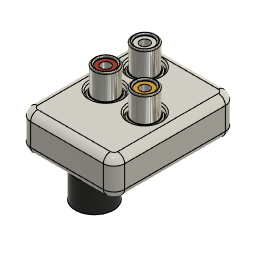
AV Adapter case v11 (Autodesk Fusion 360 design; units mm, degrees)
Autodesk Fusion 360 part; units mm, degrees
sketch "top place" plane through (0, 0, 0) normal (0, 0, 1) x (1, 0, 0) in component "PCB"
  arc A0 (28, 37) -> (27, 38) centre (27, 37) ccw
  line L0 (28, 37) -> (28, 1)
  line L1 (1, 38) -> (27, 38)
  arc A1 (27, 0) -> (28, 1) centre (27, 1) ccw
  line L2 (27, 0) -> (1, 0)
  arc A2 (0, 1) -> (1, 0) centre (1, 1) ccw
  line L3 (0, 1) -> (0, 37)
  arc A3 (1, 38) -> (0, 37) centre (1, 37) ccw
  arc A4 (25.3133, 15.5251) -> (25.3133, 20.4749) centre (21, 18) ccw
  circle A5 centre (7, 32) radius 1.7
  arc A6 (23.4749, 22.3133) -> (18.5251, 22.3133) centre (21, 18) ccw
  arc A7 (3.4645, 34.2627) -> (3.4645, 29.7373) centre (7, 32) ccw
  circle A8 centre (21, 18) radius 3.1
  arc A9 (23.2627, 21.5355) -> (18.7373, 21.5355) centre (21, 18) ccw
  arc A10 (11.3133, 29.5251) -> (11.3133, 34.4749) centre (7, 32) ccw
  arc A11 (16.6867, 20.4749) -> (16.6867, 15.5251) centre (21, 18) ccw
  arc A12 (24.5355, 15.7373) -> (24.5355, 20.2627) centre (21, 18) ccw
  arc A13 (18.5251, 13.6867) -> (23.4749, 13.6867) centre (21, 18) ccw
  arc A14 (4.5251, 27.6867) -> (9.4749, 27.6867) centre (7, 32) ccw
  arc A15 (9.4749, 36.3133) -> (4.5251, 36.3133) centre (7, 32) ccw
  arc A16 (4.7373, 28.4645) -> (9.2627, 28.4645) centre (7, 32) ccw
  circle A17 centre (7, 18) radius 3.1
  arc A18 (11.3133, 15.5251) -> (11.3133, 20.4749) centre (7, 18) ccw
  arc A19 (9.2627, 35.5355) -> (4.7373, 35.5355) centre (7, 32) ccw
  arc A20 (4.5251, 13.6867) -> (9.4749, 13.6867) centre (7, 18) ccw
  arc A21 (2.6867, 34.4749) -> (2.6867, 29.5251) centre (7, 32) ccw
  arc A22 (4.7373, 14.4645) -> (9.2627, 14.4645) centre (7, 18) ccw
  arc A23 (10.5355, 29.7373) -> (10.5355, 34.2627) centre (7, 32) ccw
  arc A24 (18.7373, 14.4645) -> (23.2627, 14.4645) centre (21, 18) ccw
  arc A25 (3.4645, 20.2627) -> (3.4645, 15.7373) centre (7, 18) ccw
  circle A26 centre (7, 32) radius 3.1
  arc A27 (17.4645, 20.2627) -> (17.4645, 15.7373) centre (21, 18) ccw
  circle A28 centre (21, 18) radius 1.7
  circle A29 centre (7, 18) radius 1.7
  arc A30 (9.2627, 21.5355) -> (4.7373, 21.5355) centre (7, 18) ccw
  arc A31 (9.4749, 22.3133) -> (4.5251, 22.3133) centre (7, 18) ccw
  arc A32 (2.6867, 20.4749) -> (2.6867, 15.5251) centre (7, 18) ccw
  arc A33 (10.5355, 15.7373) -> (10.5355, 20.2627) centre (7, 18) ccw
  arc A34 (4.7373, 21.5355) -> (3.4645, 20.2627) centre (7, 18) ccw
  arc A35 (10.5355, 20.2627) -> (9.2627, 21.5355) centre (7, 18) ccw
  arc A36 (17.4645, 15.7373) -> (18.7373, 14.4645) centre (21, 18) ccw
  arc A37 (9.4749, 27.6867) -> (11.3133, 29.5251) centre (7, 32) ccw
  arc A38 (25.3133, 20.4749) -> (23.4749, 22.3133) centre (21, 18) ccw
  arc A39 (4.7373, 35.5355) -> (3.4645, 34.2627) centre (7, 32) ccw
  arc A40 (16.6867, 15.5251) -> (18.5251, 13.6867) centre (21, 18) ccw
  arc A41 (9.2627, 14.4645) -> (10.5355, 15.7373) centre (7, 18) ccw
  arc A42 (2.6867, 29.5251) -> (4.5251, 27.6867) centre (7, 32) ccw
  arc A43 (23.4749, 13.6867) -> (25.3133, 15.5251) centre (21, 18) ccw
  arc A44 (18.5251, 22.3133) -> (16.6867, 20.4749) centre (21, 18) ccw
  arc A45 (4.5251, 22.3133) -> (2.6867, 20.4749) centre (7, 18) ccw
  arc A46 (3.4645, 29.7373) -> (4.7373, 28.4645) centre (7, 32) ccw
  arc A47 (18.7373, 21.5355) -> (17.4645, 20.2627) centre (21, 18) ccw
  arc A48 (23.2627, 14.4645) -> (24.5355, 15.7373) centre (21, 18) ccw
  arc A49 (11.3133, 20.4749) -> (9.4749, 22.3133) centre (7, 18) ccw
  arc A50 (9.2627, 28.4645) -> (10.5355, 29.7373) centre (7, 32) ccw
  arc A51 (10.5355, 34.2627) -> (9.2627, 35.5355) centre (7, 32) ccw
  arc A52 (9.4749, 13.6867) -> (11.3133, 15.5251) centre (7, 18) ccw
  arc A53 (11.3133, 34.4749) -> (9.4749, 36.3133) centre (7, 32) ccw
  arc A54 (2.6867, 15.5251) -> (4.5251, 13.6867) centre (7, 18) ccw
  arc A55 (24.5355, 20.2627) -> (23.2627, 21.5355) centre (21, 18) ccw
  arc A56 (4.5251, 36.3133) -> (2.6867, 34.4749) centre (7, 32) ccw
  arc A57 (3.4645, 15.7373) -> (4.7373, 14.4645) centre (7, 18) ccw
extrude "Extrude1" add sketch "top place" against normal blind 1.6 contours A0 L0 L1 A1 L2 A2 L3 A3 | A4 A6 A11 A13 A38 A40 A43 A44 | A5 | A7 A16 A19 A23 A39 A46 A50 A51 | A8 | A9 A12 A24 A27 A36 A47 A48 A55 | A10 A14 A15 A21 A37 A42 A53 A56 | A17 | A18 A20 A31 A32 A45 A49 A52 A54 | A22 A25 A30 A33 A34 A35 A41 A57 | A26 | A28 | A29 makes body 1 in component "PCB"
extrude "Extrude2" add sketch "top place" along normal blind 16.3 contours A8 | A17 | A26 bodies 1 in component "PCB"
extrude "Extrude3" add sketch "top place" along normal blind 17 contours A7 A16 A19 A23 A39 A46 A50 A51 | A9 A12 A24 A27 A36 A47 A48 A55 | A22 A25 A30 A33 A34 A35 A41 A57 bodies 1 in component "PCB"
extrude "Extrude4" add sketch "top place" along normal blind 8 contours A4 A6 A11 A13 A38 A40 A43 A44 | A10 A14 A15 A21 A37 A42 A53 A56 | A18 A20 A31 A32 A45 A49 A52 A54 bodies 1 in component "PCB"
fillet "Fillet2" radius 0.5 9 edges at (10.1265, 21.8671, 8) (9.478, 21.3881, 17) (4.1098, 19.121, 17) (10.8671, 28.8735, 8) (4.522, 28.6119, 17) (4.1098, 33.121, 17) (24.8671, 14.8735, 8) (18.522, 14.6119, 17) (18.1098, 19.121, 17) on bodies 1 in component "PCB"
ref_plane "WorkPlane1" through (0, 0, -1.6) normal (0, 0, 1) x (1, 0, 0) in component "PCB"
sketch "bottom place" plane through (0, 0, -1.6) normal (0, 0, 1) x (1, 0, 0) in component "PCB"
  arc A0 (28, 37) -> (27, 38) centre (27, 37) ccw
  line L0 (27, 0) -> (1, 0)
  arc A1 (27, 0) -> (28, 1) centre (27, 1) ccw
  arc A2 (0, 1) -> (1, 0) centre (1, 1) ccw
  line L1 (0, 1) -> (0, 37)
  line L2 (28, 37) -> (28, 1)
  arc A3 (1, 38) -> (0, 37) centre (1, 37) ccw
  line L3 (1, 38) -> (27, 38)
  circle A4 centre (13, 8) radius 6.8
  arc A5 (11.9, 14.1) -> (14.1, 14.1) centre (13, 14.2) ccw
  circle A6 centre (13, 8) radius 6.2
  circle A7 centre (16.5, 8) radius 0.8
  circle A8 centre (9.5, 8) radius 0.8
  circle A9 centre (15.47, 5.53) radius 0.8
  circle A10 centre (13, 4.5) radius 0.8
  circle A11 centre (10.53, 5.53) radius 0.8
extrude "Extrude5" add sketch "bottom place" against normal blind 14.51 contours A7 | A8 | A9 | A10 | A11 bodies 1 in component "PCB"
chamfer "Chamfer1" distance 0.5 angle 45 5 edges at (15.7541, 8.2893, -16.11) (14.7241, 5.8193, -16.11) (12.2541, 4.7893, -16.11) (9.7841, 5.8193, -16.11) (8.7541, 8.2893, -16.11) on bodies 1 in component "PCB"
extrude "Extrude6" add sketch "bottom place" against normal blind 3 from surface at -3 contours A5 A6 | A5 A6 bodies 1 in component "PCB"
extrude "Extrude7" add sketch "bottom place" against normal blind 10 from surface at -5.5 contours A4 bodies 1 in component "PCB"
sketch "bottom stop mask" plane through (0, 0, -1.6) normal (0, 0, 1) x (1, 0, 0) in component "PCB"
  line L0 (27, 0) -> (1, 0)
  arc A0 (27, 0) -> (28, 1) centre (27, 1) ccw
  line L1 (0, 1) -> (0, 37)
  arc A1 (28, 37) -> (27, 38) centre (27, 37) ccw
  line L2 (1, 38) -> (27, 38)
  arc A2 (1, 38) -> (0, 37) centre (1, 37) ccw
  line L3 (28, 37) -> (28, 1)
  arc A3 (0, 1) -> (1, 0) centre (1, 1) ccw
  line L4 (14.5294, 4.5894) -> (16.4106, 2.7082)
  circle A4 centre (24.5355, 21.5355) radius 1.3716
  arc A5 (16.4106, 2.7082) -> (18.2918, 4.5894) centre (17.3512, 3.6488) ccw
  line L5 (9.5, 9.3302) -> (6.8396, 9.3302)
  arc A6 (16.5, 9.3302) -> (16.5, 6.6698) centre (16.5, 8) ccw
  arc A7 (9.5, 6.6698) -> (9.5, 9.3302) centre (9.5, 8) ccw
  line L6 (14.3302, 1.8396) -> (14.3302, 4.5)
  line L7 (16.5, 6.6698) -> (19.1604, 6.6698)
  circle A8 centre (17.4645, 21.5355) radius 1.3716
  circle A9 centre (24.5355, 14.4645) radius 1.3716
  arc A10 (19.1604, 6.6698) -> (19.1604, 9.3302) centre (19.1604, 8) ccw
  line L8 (11.6698, 4.5) -> (11.6698, 1.8396)
  line L9 (6.8396, 6.6698) -> (9.5, 6.6698)
  line L10 (19.1604, 9.3302) -> (16.5, 9.3302)
  arc A11 (6.8396, 9.3302) -> (6.8396, 6.6698) centre (6.8396, 8) ccw
  arc A12 (11.6698, 1.8396) -> (14.3302, 1.8396) centre (13, 1.8396) ccw
  line L11 (9.5894, 6.4706) -> (7.7082, 4.5894)
  arc A13 (14.3302, 4.5) -> (11.6698, 4.5) centre (13, 4.5) ccw
  circle A14 centre (3.4645, 28.4645) radius 1.3716
  circle A15 centre (3.4645, 21.5355) radius 1.3716
  circle A16 centre (10.5355, 28.4645) radius 1.3716
  circle A17 centre (10.5355, 21.5355) radius 1.3716
  circle A18 centre (7, 18) radius 1.1938
  arc A19 (7.7082, 4.5894) -> (9.5894, 2.7082) centre (8.6488, 3.6488) ccw
  circle A20 centre (10.5355, 35.5355) radius 1.3716
  circle A21 centre (17.4645, 14.4645) radius 1.3716
  circle A22 centre (21, 18) radius 1.1938
  line L12 (18.2918, 4.5894) -> (16.4106, 6.4706)
  arc A23 (16.4106, 6.4706) -> (14.5294, 4.5894) centre (15.47, 5.53) ccw
  circle A24 centre (10.5355, 14.4645) radius 1.3716
  arc A25 (11.4706, 4.5894) -> (9.5894, 6.4706) centre (10.53, 5.53) ccw
  line L13 (9.5894, 2.7082) -> (11.4706, 4.5894)
  circle A26 centre (7, 32) radius 1.1938
  circle A27 centre (3.4645, 14.4645) radius 1.3716
  circle A28 centre (3.4645, 35.5355) radius 1.3716
extrude "Extrude8" add sketch "bottom stop mask" against normal blind 1.5 contours A4 | A8 | A9 | A14 | A15 | A16 | A17 | A18 | A20 | A21 | A22 | A24 | A26 | A27 | A28 bodies 1 in component "PCB"
chamfer "Chamfer2" distance 0.5 angle 45 15 edges at (23.2567, 22.0315, -3.1) (23.2567, 14.9605, -3.1) (19.887, 18.4317, -3.1) (16.1857, 22.0315, -3.1) (16.1857, 14.9605, -3.1) (9.2567, 14.9605, -3.1) (9.2567, 22.0315, -3.1) (9.2567, 28.9605, -3.1) (9.2567, 36.0315, -3.1) (5.887, 32.4317, -3.1) (2.1857, 36.0315, -3.1) (2.1857, 28.9605, -3.1) (2.1857, 22.0315, -3.1) (5.887, 18.4317, -3.1) (2.1857, 14.9605, -3.1) on bodies 1 in component "PCB"
ref_plane "WorkPlane1" through (14, 19, -1.7) normal (0, 0, -1) x (-1, 0, 0) in component "bottom shell"
sketch "bottom shell base" plane through (14, 19, -1.7) normal (0, 0, -1) x (1, 0, 0) in component "bottom shell"
  line L0 (-13, -19) -> (13, -19) construction
  arc A0 (-14, -18) -> (-13, -19) centre (-13, -18) ccw construction
  line L1 (-14, 18) -> (-14, -18) construction
  arc A1 (-13, 19) -> (-14, 18) centre (-13, 18) ccw construction
  line L2 (13, 19) -> (-13, 19) construction
  arc A2 (14, 18) -> (13, 19) centre (13, 18) ccw construction
  line L3 (14, -18) -> (14, 18) construction
  arc A3 (13, -19) -> (14, -18) centre (13, -18) ccw construction
  circle A4 centre (-1, 11) radius 6.8 construction
  line L4 (-14.3, 18) -> (-14.3, -18)
  arc A5 (-14.3, -18) -> (-13, -19.3) centre (-13, -18) ccw
  line L5 (-13, -19.3) -> (13, -19.3)
  arc A6 (13, -19.3) -> (14.3, -18) centre (13, -18) ccw
  line L6 (14.3, -18) -> (14.3, 18)
  arc A7 (14.3, 18) -> (13, 19.3) centre (13, 18) ccw
  line L7 (13, 19.3) -> (-13, 19.3)
  arc A8 (-13, 19.3) -> (-14.3, 18) centre (-13, 18) ccw
  circle A9 centre (-1, 11) radius 7.1
  line L8 (-13, -21.8) -> (13, -21.8)
  arc A10 (13, -21.8) -> (16.8, -18) centre (13, -18) ccw
  line L9 (16.8, -18) -> (16.8, 18)
  arc A11 (16.8, 18) -> (13, 21.8) centre (13, 18) ccw
  line L10 (13, 21.8) -> (-13, 21.8)
  arc A12 (-13, 21.8) -> (-16.8, 18) centre (-13, 18) ccw
  line L11 (-16.8, 18) -> (-16.8, -18)
  arc A13 (-16.8, -18) -> (-13, -21.8) centre (-13, -18) ccw
  line L12 (-13, -20.8) -> (13, -20.8)
  arc A14 (13, -20.8) -> (15.8, -18) centre (13, -18) ccw
  line L13 (15.8, -18) -> (15.8, 18)
  arc A15 (15.8, 18) -> (13, 20.8) centre (13, 18) ccw
  line L14 (13, 20.8) -> (-13, 20.8)
  arc A16 (-13, 20.8) -> (-15.8, 18) centre (-13, 18) ccw
  line L15 (-15.8, 18) -> (-15.8, -18)
  arc A17 (-15.8, -18) -> (-13, -20.8) centre (-13, -18) ccw
  dimension "d27" = 0.3
  dimension "d28" = 0.3
  dimension "d31" = 2.8
  dimension "d32" = 1.8
extrude "Extrude1'" add sketch "bottom shell base" along normal blind 2.5 separate body contours L4 A5 L5 A6 L6 A7 L7 A8 | L8 A10 L9 A11 L10 A12 L11 A13 | L12 A14 L13 A15 L14 A16 L15 A17 makes body 2 in component "bottom shell"
sketch "solder pads" plane through (0, 0, -1.7) normal (0, 0, 1) x (-1, 0, 0) in component "bottom shell"
  circle A0 centre (-13, -8) radius 7.1
  arc A1 (-1, -40.8) -> (2.8, -37) centre (-1, -37) ccw
  line L0 (2.8, -37) -> (2.8, -1)
  arc A2 (2.8, -1) -> (-1, 2.8) centre (-1, -1) ccw
  line L1 (-1, 2.8) -> (-27, 2.8)
  arc A3 (-27, 2.8) -> (-30.8, -1) centre (-27, -1) ccw
  line L2 (-30.8, -1) -> (-30.8, -37)
  arc A4 (-30.8, -37) -> (-27, -40.8) centre (-27, -37) ccw
  line L3 (-27, -40.8) -> (-1, -40.8)
  circle A5 centre (-3.4645, -14.4645) radius 1.3716 construction
  circle A6 centre (-3.4645, -21.5355) radius 1.3716 construction
  circle A7 centre (-7, -18) radius 1.1938 construction
  circle A8 centre (-10.5355, -14.4645) radius 1.3716 construction
  circle A9 centre (-10.5355, -21.5355) radius 1.3716 construction
  circle A10 centre (-10.5355, -28.4645) radius 1.3716 construction
  circle A11 centre (-10.5355, -35.5355) radius 1.3716 construction
  circle A12 centre (-3.4645, -35.5355) radius 1.3716 construction
  circle A13 centre (-3.4645, -28.4645) radius 1.3716 construction
  circle A14 centre (-7, -32) radius 1.1938 construction
  circle A15 centre (-7, -32) radius 1.1938 construction
  circle A16 centre (-17.4645, -21.5355) radius 1.3716 construction
  circle A17 centre (-24.5355, -21.5355) radius 1.3716 construction
  circle A18 centre (-21, -18) radius 1.1938 construction
  circle A19 centre (-24.5355, -14.4645) radius 1.3716 construction
  circle A20 centre (-17.4645, -14.4645) radius 1.3716 construction
  circle A21 centre (-17.4645, -14.4645) radius 1.3716 construction
  circle A22 centre (-24.5355, -14.4645) radius 1.8716
  circle A23 centre (-24.5355, -21.5355) radius 1.8716
  circle A24 centre (-21, -18) radius 1.6938
  circle A25 centre (-17.4645, -14.4645) radius 1.8716
  circle A26 centre (-17.4645, -21.5355) radius 1.8716
  circle A27 centre (-10.5355, -14.4645) radius 1.8716
  circle A28 centre (-10.5355, -21.5355) radius 1.8716
  circle A29 centre (-7, -18) radius 1.6938
  circle A30 centre (-3.4645, -14.4645) radius 1.8716
  circle A31 centre (-3.4645, -21.5355) radius 1.8716
  circle A32 centre (-3.4645, -28.4645) radius 1.8716
  circle A33 centre (-10.5355, -28.4645) radius 1.8716
  circle A34 centre (-10.5355, -35.5355) radius 1.8716
  circle A35 centre (-7, -32) radius 1.6938
  circle A36 centre (-3.4645, -35.5355) radius 1.8716
  dimension "d35" = 0.5
  dimension "d36" = 0.5
  dimension "d37" = 0.5
  dimension "d38" = 0.5
  dimension "d39" = 0.5
  dimension "d40" = 0.5
  dimension "d41" = 0.5
  dimension "d42" = 0.5
  dimension "d43" = 0.5
  dimension "d44" = 0.5
  dimension "d45" = 0.5
  dimension "d46" = 0.5
  dimension "d47" = 0.5
  dimension "d48" = 0.5
  dimension "d49" = 0.5
extrude "Extrude2'" cut sketch "solder pads" against normal blind 1.5 contours A0 A25 | A0 A27 | A22 | A23 | A24 | A26 | A28 | A29 | A30 | A31 | A32 | A33 | A34 | A35 | A36 picked at (-16.7645, -14.7878) picked at (-9.7455, -14.867) bodies 2 in component "bottom shell"
extrude "Extrude3'" add sketch "bottom shell base" against normal blind 6.5 contours L12 A14 L13 A15 L14 A16 L15 A17 bodies 2 in component "bottom shell"
extrude "Extrude4'" add sketch "bottom shell base" against normal blind 8 contours L8 A10 L9 A11 L10 A12 L11 A13 bodies 2 in component "bottom shell"
fillet "Fillet1" radius 2.5 8 edges at (14, 40.8, -4.2) (29.687, 39.687, -4.2) (30.8, 19, -4.2) (29.687, -1.687, -4.2) (14, -2.8, -4.2) (-1.687, -1.687, -4.2) (-2.8, 19, -4.2) (-1.687, 39.687, -4.2) on bodies 2 in component "bottom shell"
ref_plane "WorkPlane1" through (29.8, -2.8, 6.3) normal (0, 0, 1) x (1, 0, 0) in component "top shell"
sketch "top shell" plane through (29.5, -2.3, 6.3) normal (0, 0, 1) x (1, 0, 0) in component "top shell"
  arc A0 (-32.3, 3.3) -> (-28.5, -0.5) centre (-28.5, 3.3) ccw
  line L0 (-32.3, 39.3) -> (-32.3, 3.3)
  arc A1 (-28.5, 43.1) -> (-32.3, 39.3) centre (-28.5, 39.3) ccw
  line L1 (-2.5, 43.1) -> (-28.5, 43.1)
  arc A2 (1.3, 39.3) -> (-2.5, 43.1) centre (-2.5, 39.3) ccw
  line L2 (1.3, 3.3) -> (1.3, 39.3)
  arc A3 (-2.5, -0.5) -> (1.3, 3.3) centre (-2.5, 3.3) ccw
  line L3 (-28.5, -0.5) -> (-2.5, -0.5)
  line L4 (-29.8, 3.3) -> (-29.8, 39.3)
  arc A4 (-29.8, 3.3) -> (-28.5, 2) centre (-28.5, 3.3) ccw
  line L5 (-2.5, 2) -> (-28.5, 2)
  arc A5 (-28.5, 40.6) -> (-29.8, 39.3) centre (-28.5, 39.3) ccw
  line L6 (-28.5, 40.6) -> (-2.5, 40.6)
  arc A6 (-1.2, 39.3) -> (-2.5, 40.6) centre (-2.5, 39.3) ccw
  line L7 (-1.2, 39.3) -> (-1.2, 3.3)
  arc A7 (-2.5, 2) -> (-1.2, 3.3) centre (-2.5, 3.3) ccw
  arc A8 (-26.8133, 36.7749) -> (-26.8133, 31.8251) centre (-22.5, 34.3) ccw construction
  arc A9 (-26.8133, 31.8251) -> (-24.9749, 29.9867) centre (-22.5, 34.3) ccw construction
  arc A10 (-24.9749, 29.9867) -> (-20.0251, 29.9867) centre (-22.5, 34.3) ccw construction
  arc A11 (-20.0251, 29.9867) -> (-18.1867, 31.8251) centre (-22.5, 34.3) ccw construction
  arc A12 (-18.1867, 31.8251) -> (-18.1867, 36.7749) centre (-22.5, 34.3) ccw construction
  arc A13 (-18.1867, 36.7749) -> (-20.0251, 38.6133) centre (-22.5, 34.3) ccw construction
  arc A14 (-20.0251, 38.6133) -> (-24.9749, 38.6133) centre (-22.5, 34.3) ccw construction
  arc A15 (-24.9749, 38.6133) -> (-26.8133, 36.7749) centre (-22.5, 34.3) ccw construction
  arc A16 (-24.9749, 24.6133) -> (-26.8133, 22.7749) centre (-22.5, 20.3) ccw construction
  arc A17 (-20.0251, 24.6133) -> (-24.9749, 24.6133) centre (-22.5, 20.3) ccw construction
  arc A18 (-18.1867, 22.7749) -> (-20.0251, 24.6133) centre (-22.5, 20.3) ccw construction
  arc A19 (-18.1867, 17.8251) -> (-18.1867, 22.7749) centre (-22.5, 20.3) ccw construction
  arc A20 (-20.0251, 15.9867) -> (-18.1867, 17.8251) centre (-22.5, 20.3) ccw construction
  arc A21 (-24.9749, 15.9867) -> (-20.0251, 15.9867) centre (-22.5, 20.3) ccw construction
  arc A22 (-26.8133, 17.8251) -> (-24.9749, 15.9867) centre (-22.5, 20.3) ccw construction
  arc A23 (-26.8133, 22.7749) -> (-26.8133, 17.8251) centre (-22.5, 20.3) ccw construction
  arc A24 (-10.9749, 24.6133) -> (-12.8133, 22.7749) centre (-8.5, 20.3) ccw construction
  arc A25 (-12.8133, 22.7749) -> (-12.8133, 17.8251) centre (-8.5, 20.3) ccw construction
  arc A26 (-12.8133, 17.8251) -> (-10.9749, 15.9867) centre (-8.5, 20.3) ccw construction
  arc A27 (-10.9749, 15.9867) -> (-6.0251, 15.9867) centre (-8.5, 20.3) ccw construction
  arc A28 (-6.0251, 15.9867) -> (-4.1867, 17.8251) centre (-8.5, 20.3) ccw construction
  arc A29 (-4.1867, 17.8251) -> (-4.1867, 22.7749) centre (-8.5, 20.3) ccw construction
  arc A30 (-4.1867, 22.7749) -> (-6.0251, 24.6133) centre (-8.5, 20.3) ccw construction
  arc A31 (-6.0251, 24.6133) -> (-10.9749, 24.6133) centre (-8.5, 20.3) ccw construction
  arc A32 (-19.7763, 15.553) -> (-17.753, 17.5763) centre (-22.5, 20.3) ccw
  arc A33 (-17.753, 17.5763) -> (-17.753, 23.0237) centre (-22.5, 20.3) ccw
  arc A34 (-17.753, 23.0237) -> (-19.7763, 25.047) centre (-22.5, 20.3) ccw
  arc A35 (-19.7763, 25.047) -> (-25.2237, 25.047) centre (-22.5, 20.3) ccw
  arc A36 (-25.2237, 25.047) -> (-27.247, 23.0237) centre (-22.5, 20.3) ccw
  arc A37 (-27.247, 23.0237) -> (-27.247, 17.5763) centre (-22.5, 20.3) ccw
  arc A38 (-27.247, 17.5763) -> (-25.2237, 15.553) centre (-22.5, 20.3) ccw
  arc A39 (-25.2237, 15.553) -> (-19.7763, 15.553) centre (-22.5, 20.3) ccw
  arc A40 (-19.7763, 39.047) -> (-25.2237, 39.047) centre (-22.5, 34.3) ccw
  arc A41 (-25.2237, 39.047) -> (-27.247, 37.0237) centre (-22.5, 34.3) ccw
  arc A42 (-27.247, 37.0237) -> (-27.247, 31.5763) centre (-22.5, 34.3) ccw
  arc A43 (-27.247, 31.5763) -> (-25.2237, 29.553) centre (-22.5, 34.3) ccw
  arc A44 (-25.2237, 29.553) -> (-19.7763, 29.553) centre (-22.5, 34.3) ccw
  arc A45 (-19.7763, 29.553) -> (-17.753, 31.5763) centre (-22.5, 34.3) ccw
  arc A46 (-17.753, 31.5763) -> (-17.753, 37.0237) centre (-22.5, 34.3) ccw
  arc A47 (-17.753, 37.0237) -> (-19.7763, 39.047) centre (-22.5, 34.3) ccw
  arc A48 (-5.7763, 15.553) -> (-3.753, 17.5763) centre (-8.5, 20.3) ccw
  arc A49 (-3.753, 17.5763) -> (-3.753, 23.0237) centre (-8.5, 20.3) ccw
  arc A50 (-3.753, 23.0237) -> (-5.7763, 25.047) centre (-8.5, 20.3) ccw
  arc A51 (-5.7763, 25.047) -> (-11.2237, 25.047) centre (-8.5, 20.3) ccw
  arc A52 (-11.2237, 25.047) -> (-13.247, 23.0237) centre (-8.5, 20.3) ccw
  arc A53 (-13.247, 23.0237) -> (-13.247, 17.5763) centre (-8.5, 20.3) ccw
  arc A54 (-13.247, 17.5763) -> (-11.2237, 15.553) centre (-8.5, 20.3) ccw
  arc A55 (-11.2237, 15.553) -> (-5.7763, 15.553) centre (-8.5, 20.3) ccw
  arc A56 (-28.5, 41.6) -> (-30.8, 39.3) centre (-28.5, 39.3) ccw
  line L8 (-30.8, 3.3) -> (-30.8, 39.3)
  arc A57 (-30.8, 3.3) -> (-28.5, 1) centre (-28.5, 3.3) ccw
  line L9 (-2.5, 1) -> (-28.5, 1)
  arc A58 (-2.5, 1) -> (-0.2, 3.3) centre (-2.5, 3.3) ccw
  line L10 (-0.2, 39.3) -> (-0.2, 3.3)
  arc A59 (-0.2, 39.3) -> (-2.5, 41.6) centre (-2.5, 39.3) ccw
  line L11 (-28.5, 41.6) -> (-2.5, 41.6)
  circle A60 centre (-16.5, 10.3) radius 6.8 construction
  circle A61 centre (-16.5, 10.3) radius 2
  line L12 (-29.8, 6) -> (-27.3, 6)
  line L13 (-27.3, 6) -> (-27.3, 14)
  line L14 (-27.3, 14) -> (-29.8, 14)
  line L15 (-29.8, 14) -> (-29.8, 6)
  line L16 (-9.7, 2) -> (-17.7, 2)
  line L17 (-17.7, 2) -> (-17.7, 4.5)
  line L18 (-17.7, 4.5) -> (-9.7, 4.5)
  line L19 (-9.7, 4.5) -> (-9.7, 2)
  line L20 (-17.7, 40.6) -> (-9.7, 40.6)
  line L21 (-9.7, 40.6) -> (-9.7, 38.1)
  line L22 (-9.7, 38.1) -> (-17.7, 38.1)
  line L23 (-17.7, 38.1) -> (-17.7, 40.6)
  line L24 (-1.2, 14) -> (-3.7, 14)
  line L25 (-3.7, 14) -> (-3.7, 6)
  line L26 (-3.7, 6) -> (-1.2, 6)
  line L27 (-1.2, 6) -> (-1.2, 14)
  circle A62 centre (-10.2, 32.6) radius 2
  dimension "d61" = 0.5
  dimension "d62" = 0.5
  dimension "d63" = 0.5
  dimension "d64" = 1
  dimension "d65" = 4
  dimension "d69" = 2.5
  dimension "d70" = 8
  dimension "d71" = 4
  dimension "d72" = 8
  dimension "d73" = 2.5
  dimension "d74" = 8.5
  dimension "d75" = 8
  dimension "d76" = 2.5
  dimension "d78" = 2.5
  dimension "d79" = 8
  dimension "d81" = 4
  dimension "d82" = 9
  dimension "d83" = 9
  constraint concentric A60 A61
  constraint horizontal L12
  constraint vertical L13
  constraint horizontal L14
  constraint vertical L15
  constraint coincident L4 L12.start
  constraint horizontal L16
  constraint vertical L17
  constraint horizontal L18
  constraint vertical L19
  constraint coincident L5 L16.start
  constraint horizontal L20
  constraint vertical L21
  constraint horizontal L22
  constraint vertical L23
  constraint coincident L6 L20.start
  constraint horizontal L24
  constraint vertical L25
  constraint horizontal L26
  constraint vertical L27
  constraint coincident L7 L24.start
  constraint collinear L14 L24
  constraint collinear L17 L23
  measures "d65" diameter of A61
  measures "d69" distance of L12.start L12.end
  measures "d70" distance of L12.start L14.end
  measures "d71" distance of L5 L12
  measures "d72" distance of L16.start L16.end
  measures "d73" distance of L16.start L18.end
  measures "d74" distance of L7 L19
  measures "d75" distance of L20.start L20.end
  measures "d76" distance of L20.start L22.end
  measures "d78" distance of L24.start L24.end
  measures "d79" distance of L24.start L26.end
  measures "d81" diameter of A62
  measures "d82" distance of L11 A62.centre
  measures "d83" distance of L7 A62.centre
extrude "Extrude1''" add sketch "top shell" along normal blind 2.5 separate body contours A0 L0 A1 L1 A2 L2 A3 L3 | L4 A4 L5 A5 L6 A6 L7 A7 L12 L13 L14 L17 L18 L19 L21 L22 L23 L24 L25 L26 | L4 L12 L13 L14 L15 | L5 L16 L17 L18 L19 | L6 L20 L21 L22 L23 | L7 L24 L25 L26 L27 | A56 L8 A57 L9 A58 L10 A59 L11 | A61 | A62 makes body 3 in component "top shell"
extrude "Extrude2''" add sketch "top shell" against normal blind 1.5 contours A56 L8 A57 L9 A58 L10 A59 L11 bodies 3 in component "top shell"
extrude "Extrude3''" add sketch "top shell" against normal blind 6 draft -7 contours A61 | A62 bodies 3 in component "top shell"
extrude "Extrude4''" add sketch "top shell" against normal blind 6 contours L4 L12 L13 L14 L15 | L5 L16 L17 L18 L19 | L6 L20 L21 L22 L23 | L7 L24 L25 L26 L27 bodies 3 in component "top shell"
sketch "bot_hook" plane through (11.8, 0, 0) normal (-1, 0, 0) x (0, -1, 0) in component "top shell"
  line L0 (0.3, 6.3) -> (-2.2, 6.3)
  line L1 (-2.2, 6.3) -> (-2.2, 0.3)
  line L2 (-2.2, 0.3) -> (0.3, 0.3)
  line L3 (0.3, 0.3) -> (0.3, 4.8)
  line L4 (0.3, 4.8) -> (0.3, 6.3)
  line L5 (0.3, 0.3) -> (-2.2, 0.3) construction
  line L6 (0.3, 4.8) -> (0.3, 0.3) construction
  line L7 (0.3, 0.3) -> (1.1, 2.7374)
  line L8 (1.1, 2.7374) -> (0.3, 3)
  line L9 (0.3, 0.3) -> (0.3, 3)
  dimension "d95" = 0.8
  dimension "d96" = 2.7
  constraint coincident L2.end L3.start
  constraint coincident L3 L8.end
  constraint perpendicular L7 L8
  measures "d95" horizontal distance of L2.end L7.end
  measures "d96" distance of L2.end L8.end
sketch "left_hook" plane through (0, 3.7, 0) normal (0, -1, 0) x (1, 0, 0) in component "top shell"
  line L0 (28.3, 6.3) -> (25.8, 6.3)
  line L1 (25.8, 6.3) -> (25.8, 0.3)
  line L2 (25.8, 0.3) -> (28.3, 0.3)
  line L3 (28.3, 0.3) -> (28.3, 4.8)
  line L4 (28.3, 4.8) -> (28.3, 6.3)
  line L5 (28.3, 0.3) -> (25.8, 0.3) construction
  line L6 (28.3, 4.8) -> (28.3, 0.3) construction
  line L7 (28.3, 0.3) -> (29.1, 2.7374)
  line L8 (29.1, 2.7374) -> (28.3, 3)
  line L9 (28.3, 3) -> (28.3, 0.3)
  dimension "d97" = 0.8
  dimension "d98" = 2.7
  constraint coincident L2.end L3.start
  constraint coincident L3 L8.end
  constraint perpendicular L7 L8
  measures "d97" distance of L3 L7.end
  measures "d98" distance of L8.end L2.end
sketch "right_hook" plane through (0, 11.7, 0) normal (0, 1, 0) x (-1, 0, 0) in component "top shell"
  line L0 (0.3, 6.3) -> (-2.2, 6.3)
  line L1 (-2.2, 6.3) -> (-2.2, 0.3)
  line L2 (-2.2, 0.3) -> (0.3, 0.3)
  line L3 (0.3, 0.3) -> (0.3, 4.8)
  line L4 (0.3, 4.8) -> (0.3, 6.3)
  line L5 (0.3, 0.3) -> (-2.2, 0.3) construction
  line L6 (0.3, 4.8) -> (0.3, 0.3) construction
  line L7 (0.3, 0.3) -> (1.1, 2.7374)
  line L8 (1.1, 2.7374) -> (0.3, 3)
  line L9 (0.3, 3) -> (0.3, 0.3)
  dimension "d99" = 2.7
  dimension "d100" = 0.8
  constraint coincident L2.end L3.start
  constraint coincident L6 L8.end
  constraint perpendicular L7 L8
  measures "d99" distance of L2.end L8.end
  measures "d100" distance of L7.end L9
sketch "top_hook" plane through (11.8, 0, 0) normal (-1, 0, 0) x (0, -1, 0) in component "top shell"
  line L0 (-35.8, 6.3) -> (-38.3, 6.3)
  line L1 (-38.3, 6.3) -> (-38.3, 4.8)
  line L2 (-38.3, 4.8) -> (-38.3, 0.3)
  line L3 (-38.3, 0.3) -> (-35.8, 0.3)
  line L4 (-35.8, 0.3) -> (-35.8, 6.3)
  line L5 (-35.8, 0.3) -> (-38.3, 0.3) construction
  line L6 (-38.3, 4.8) -> (-38.3, 0.3) construction
  line L7 (-38.3, 0.3) -> (-39.1, 2.7374)
  line L8 (-39.1, 2.7374) -> (-38.3, 3)
  line L9 (-38.3, 3) -> (-38.3, 0.3)
  dimension "d101" = 2.7
  dimension "d102" = 0.8
  constraint coincident L2.end L3.start
  constraint coincident L6 L8.end
  constraint perpendicular L7 L8
  measures "d101" distance of L8.end L2.end
  measures "d102" distance of L7.end L9
extrude "Extrude5'" add sketch "top_hook" against normal blind 8 contours L2 L7 L8 L9 bodies 3 in component "top shell"
extrude "Extrude6'" add sketch "left_hook" against normal blind 8 contours L3 L7 L8 L9 bodies 3 in component "top shell"
extrude "Extrude7'" add sketch "bot_hook" against normal blind 8 contours L3 L7 L8 L9 bodies 3 in component "top shell"
extrude "Extrude8'" add sketch "right_hook" against normal blind 8 contours L3 L7 L8 L9 bodies 3 in component "top shell"
fillet "Fillet1'" radius 2.5 8 edges at (-1.687, -1.687, 8.8) (14, -2.8, 8.8) (29.687, -1.687, 8.8) (30.8, 19, 8.8) (29.687, 39.687, 8.8) (14, 40.8, 8.8) (-1.687, 39.687, 8.8) (-2.8, 19, 8.8) on bodies 3 in component "top shell"
sketch "left" plane through (-0.3, 0, 0) normal (1, 0, 0) x (0, 1, 0) in component "bottom shell"
  line L0 (1, -1.7) -> (37, -1.7)
  line L1 (37, -1.7) -> (37, 4.8)
  line L2 (37, 4.8) -> (1, 4.8)
  line L3 (1, 4.8) -> (1, -1.7)
  line L4 (3.7, 0.3) -> (11.7, 0.3) construction
  line L5 (3.7, 6.3) -> (3.7, 0.3) construction
  line L6 (11.7, 6.3) -> (11.7, 0.3) construction
  line L7 (11.7, 0.3) -> (11.7, 2.7374) construction
  line L8 (11.7, 2.7374) -> (11.7, 3) construction
  line L9 (11.7, 3) -> (11.7, 4.8) construction
  line L10 (11.7, 4.8) -> (11.7, 6.3) construction
  line L11 (11.7, 3) -> (3.7, 3) construction
  line L12 (3.4, 6.3) -> (12, 6.3)
  line L13 (12, 6.3) -> (12, 0)
  line L14 (12, 0) -> (3.4, 0)
  line L15 (3.4, 0) -> (3.4, 6.3)
  line L16 (3.4, 3.3) -> (12, 3.3)
  dimension "d113" = 0.3
  dimension "d114" = 0.3
  dimension "d115" = 0.3
  dimension "d116" = 0.3
  constraint horizontal L12
  constraint vertical L13
  constraint horizontal L14
  constraint vertical L15
  constraint coincident L5.start L12
  constraint coincident L15 L16.start
  constraint coincident L13 L16.end
  constraint perpendicular L13 L16
  measures "d113" distance of L4 L14
  measures "d114" distance of L9 L13
  measures "d115" distance of L5 L15
  measures "d116" distance of L11 L16
sketch "bottom" plane through (0, -0.3, 0) normal (0, 1, 0) x (-1, 0, 0) in component "bottom shell"
  line L0 (-27, -1.7) -> (-1, -1.7)
  line L1 (-1, -1.7) -> (-1, 4.8)
  line L2 (-1, 4.8) -> (-27, 4.8)
  line L3 (-27, 4.8) -> (-27, -1.7)
  line L4 (-11.8, 6.3) -> (-11.8, 0.3) construction
  line L5 (-19.8, 6.3) -> (-19.8, 0.3) construction
  line L6 (-11.8, 0.3) -> (-19.8, 0.3) construction
  line L7 (-11.8, 3) -> (-19.8, 3) construction
  line L8 (-20.1, 6.3) -> (-11.5, 6.3)
  line L9 (-11.5, 6.3) -> (-11.5, 0)
  line L10 (-11.5, 0) -> (-20.1, 0)
  line L11 (-20.1, 0) -> (-20.1, 6.3)
  line L12 (-20.1, 3.3) -> (-11.5, 3.3)
  dimension "d117" = 0.3
  dimension "d118" = 0.3
  dimension "d119" = 0.3
  dimension "d120" = 0.3
  constraint horizontal L8
  constraint vertical L9
  constraint horizontal L10
  constraint vertical L11
  constraint coincident L5.start L8
  constraint coincident L11 L12.start
  constraint coincident L9 L12.end
  constraint perpendicular L9 L12
  measures "d117" distance of L6 L10
  measures "d118" distance of L4 L9
  measures "d119" distance of L5 L11
  measures "d120" distance of L7 L12
sketch "top" plane through (0, 38.3, 0) normal (0, -1, 0) x (1, 0, 0) in component "bottom shell"
  line L0 (1, -1.7) -> (27, -1.7)
  line L1 (27, -1.7) -> (27, 4.8)
  line L2 (27, 4.8) -> (1, 4.8)
  line L3 (1, 4.8) -> (1, -1.7)
  line L4 (19.8, 6.3) -> (19.8, 0.3) construction
  line L5 (19.8, 3) -> (11.8, 3) construction
  line L6 (11.8, 0.3) -> (19.8, 0.3) construction
  line L7 (11.8, 6.3) -> (11.8, 0.3) construction
  line L8 (20.1, 6.3) -> (11.5, 6.3)
  line L9 (11.5, 6.3) -> (11.5, 0)
  line L10 (11.5, 0) -> (20.1, 0)
  line L11 (20.1, 0) -> (20.1, 6.3)
  line L12 (20.1, 3.3) -> (11.5, 3.3)
  dimension "d121" = 0.3
  dimension "d122" = 0.3
  dimension "d123" = 0.3
  dimension "d124" = 0.3
  constraint horizontal L8
  constraint vertical L9
  constraint horizontal L10
  constraint vertical L11
  constraint coincident L4.start L8
  constraint coincident L11 L12.start
  constraint coincident L9 L12.end
  constraint perpendicular L9 L12
  measures "d121" distance of L5 L12
  measures "d122" distance of L6 L10
  measures "d123" distance of L4 L11
  measures "d124" distance of L7 L9
sketch "right" plane through (28.3, 0, 0) normal (-1, 0, 0) x (0, -1, 0) in component "bottom shell"
  line L0 (-37, -1.7) -> (-1, -1.7)
  line L1 (-1, -1.7) -> (-1, 4.8)
  line L2 (-1, 4.8) -> (-37, 4.8)
  line L3 (-37, 4.8) -> (-37, -1.7)
  line L4 (-11.7, 6.3) -> (-11.7, 0.3) construction
  line L5 (-11.7, 0.3) -> (-3.7, 0.3) construction
  line L6 (-3.7, 6.3) -> (-3.7, 0.3) construction
  line L7 (-3.7, 0.3) -> (-3.7, 2.7374)
  line L8 (-3.7, 2.7374) -> (-3.7, 3)
  line L9 (-3.7, 3) -> (-3.7, 4.8) construction
  line L10 (-3.7, 4.8) -> (-3.7, 6.3) construction
  line L11 (-3.7, 3) -> (-11.7, 3) construction
  line L12 (-3.4, 6.3) -> (-12, 6.3)
  line L13 (-12, 6.3) -> (-12, 0)
  line L14 (-12, 0) -> (-3.4, 0)
  line L15 (-3.4, 0) -> (-3.4, 6.3)
  line L16 (-3.4, 2.7) -> (-12, 2.7)
  dimension "d125" = 0.3
  dimension "d126" = 0.3
  dimension "d127" = 0.3
  dimension "d128" = 0.3
  constraint horizontal L12
  constraint vertical L13
  constraint horizontal L14
  constraint vertical L15
  constraint coincident L4.start L12
  constraint coincident L15 L16.start
  constraint coincident L13 L16.end
  constraint perpendicular L13 L16
  measures "d125" distance of L6 L15
  measures "d126" distance of L5 L14
  measures "d127" distance of L4 L13
  measures "d128" distance of L11 L16
extrude "Extrude5''" cut sketch "right" against normal blind 1 contours L13 L14 L15 L16 bodies 2 in component "bottom shell"
extrude "Extrude6''" cut sketch "right" against normal blind 0.2 contours L2 L13 L15 L16 bodies 2 in component "bottom shell"
extrude "Extrude7''" cut sketch "top" against normal blind 1 contours L9 L10 L11 L12 bodies 2 in component "bottom shell"
extrude "Extrude8''" cut sketch "top" against normal blind 0.2 contours L2 L9 L11 L12 bodies 2 in component "bottom shell"
extrude "Extrude9" cut sketch "left" against normal blind 1 contours L13 L14 L15 L16 bodies 2 in component "bottom shell"
extrude "Extrude10" cut sketch "left" against normal blind 0.2 contours L2 L13 L15 L16 bodies 2 in component "bottom shell"
extrude "Extrude11" cut sketch "bottom" against normal blind 1 contours L9 L10 L11 L12 bodies 2 in component "bottom shell"
extrude "Extrude12" cut sketch "bottom" against normal blind 0.2 contours L2 L9 L11 L12 bodies 2 in component "bottom shell"
fillet "Fillet2'" radius 0.5 15 edges at (5.2094, 13.7877, -3.2) (5.2094, 20.8587, -3.2) (5.2094, 27.7877, -3.2) (5.2094, 34.8587, -3.2) (8.5792, 31.3875, -3.2) (12.2804, 34.8587, -3.2) (12.2804, 27.7877, -3.2) (12.2804, 20.8587, -3.2) (8.5792, 17.3875, -3.2) (9.8688, 16.2133, -3.2) (18.5281, 16.0045, -3.2) (19.2094, 20.8587, -3.2) (22.5792, 17.3875, -3.2) (26.2804, 20.8587, -3.2) (26.2804, 13.7877, -3.2) on bodies 2 in component "bottom shell"
fillet "Fillet3" radius 0.5 17 edges at (5.2094, 13.7877, -1.7) (12.2794, 0.9367, -1.7) (9.8688, 16.2133, -1.7) (13.9803, 15.032, -1.7) (18.5281, 16.0045, -1.7) (19.2094, 20.8587, -1.7) (12.2804, 20.8587, -1.7) (8.5792, 17.3875, -1.7) (22.5792, 17.3875, -1.7) (26.2804, 20.8587, -1.7) (26.2804, 13.7877, -1.7) (12.2804, 27.7877, -1.7) (8.5792, 31.3875, -1.7) (12.2804, 34.8587, -1.7) (5.2094, 20.8587, -1.7) (5.2094, 27.7877, -1.7) (5.2094, 34.8587, -1.7) on bodies 2 in component "bottom shell"
fillet "Fillet4" radius 0.5 8 edges at (28.3, 19, -1.7) (27.9192, 37.9192, -1.7) (14, 38.3, -1.7) (0.0808, 37.9192, -1.7) (-0.3, 19, -1.7) (0.0808, 0.0808, -1.7) (14, -0.3, -1.7) (27.9192, 0.0808, -1.7) on bodies 2 in component "bottom shell"
fillet "Fillet2''" radius 0.5 24 edges at (2.2, 7.7, 6.3) (0.95, 11.7, 6.3) (-0.3, 24.35, 6.3) (0.0808, 37.9192, 6.3) (6.4, 38.3, 6.3) (0.95, 3.7, 6.3) (6.4, -0.3, 6.3) (0.0808, 0.0808, 6.3) (-0.3, 2.35, 6.3) (11.8, 0.95, 6.3) (15.8, 2.2, 6.3) (19.8, 0.95, 6.3) (28.3, 2.35, 6.3) (27.9192, 0.0808, 6.3) (23.4, -0.3, 6.3) (27.05, 3.7, 6.3) (25.8, 7.7, 6.3) (27.05, 11.7, 6.3) (23.4, 38.3, 6.3) (27.9192, 37.9192, 6.3) (28.3, 24.35, 6.3) (19.8, 37.05, 6.3) (15.8, 35.8, 6.3) (11.8, 37.05, 6.3) on bodies 3 in component "top shell"
fillet "Fillet3'" radius 0.5 2 edges at (17.4353, 29.5768, 6.3) (11.1353, 7.2768, 6.3) on bodies 3 in component "top shell"
fillet "Fillet4'" radius 0.5 3 edges at (7.8228, 12.5893, 6.3) (11.256, 35.4408, 6.3) (21.8228, 12.5893, 6.3) on bodies 3 in component "top shell"
fillet "Fillet5" radius 0.5 3 edges at (11.256, 35.4408, 8.8) (7.8228, 12.5893, 8.8) (21.8228, 12.5893, 8.8) on bodies 3 in component "top shell"
sketch "label outline" plane through (0, 0, 8.8) normal (0, 0, 1) x (-1, 0, 0) in component "top shell"
  circle A0 centre (-7, -18) radius 5.9729
  arc A1 (0.3, -1) -> (-1, 0.3) centre (-1, -1) ccw
  line L0 (-1, 0.3) -> (-27, 0.3)
  arc A2 (-27, 0.3) -> (-28.3, -1) centre (-27, -1) ccw
  line L1 (-28.3, -1) -> (-28.3, -37)
  arc A3 (-28.3, -37) -> (-27, -38.3) centre (-27, -37) ccw
  line L2 (-27, -38.3) -> (-1, -38.3)
  arc A4 (-1, -38.3) -> (0.3, -37) centre (-1, -37) ccw
  line L3 (0.3, -37) -> (0.3, -1)
  circle A5 centre (-7, -32) radius 5.9729
  circle A6 centre (-21, -18) radius 5.9729
  circle A7 centre (-7, -32) radius 5.4729
  circle A8 centre (-7, -18) radius 5.4729
  circle A9 centre (-21, -18) radius 5.4729
  line L4 (0.3, -1) -> (0.3, -37) construction
  arc A10 (-1, -38.3) -> (0.3, -37) centre (-1, -37) ccw construction
  line L5 (-1, -38.3) -> (-27, -38.3) construction
  arc A11 (-28.3, -37) -> (-27, -38.3) centre (-27, -37) ccw construction
  line L6 (-28.3, -37) -> (-28.3, -1) construction
  arc A12 (-27, 0.3) -> (-28.3, -1) centre (-27, -1) ccw construction
  line L7 (-27, 0.3) -> (-1, 0.3) construction
  arc A13 (0.3, -1) -> (-1, 0.3) centre (-1, -1) ccw construction
  arc A14 (-28.8, -37) -> (-27, -38.8) centre (-27, -37) ccw
  line L8 (-1, -38.8) -> (-27, -38.8)
  arc A15 (-1, -38.8) -> (0.8, -37) centre (-1, -37) ccw
  line L9 (0.8, -1) -> (0.8, -37)
  arc A16 (0.8, -1) -> (-1, 0.8) centre (-1, -1) ccw
  line L10 (-27, 0.8) -> (-1, 0.8)
  arc A17 (-27, 0.8) -> (-28.8, -1) centre (-27, -1) ccw
  line L11 (-28.8, -37) -> (-28.8, -1)
  dimension "d162" = -0.5
component "PCB" placed x (1, 0, 0) y (0, 1, 0) z (0, 0, 1) at (0, 0, 0)
component "bottom shell" placed x (1, 0, 0) y (0, 1, 0) z (0, 0, 1) at (0, 0, 0)
component "top shell" placed x (1, 0, 0) y (0, 1, 0) z (0, 0, 1) at (0, 0, 0)
equation "d27 = tol"
equation "d28 = tol"
equation "tol = 0.3 mm"
equation "wall = 2.5 mm"
equation "d31 = wall + tol"
equation "d32 = tol + 0.6 * wall"
equation "d33 = wall"
equation "pad_depression = 1.5 mm"
equation "d51 = -pad_depression"
equation "bottom_height = 8 mm"
equation "overlap = 1.5 mm"
equation "d55 = -bottom_height + overlap"
equation "d57 = -bottom_height"
equation "d60 = wall"
equation "d61 = tol_rad"
equation "d62 = tol_rad"
equation "d63 = tol_rad"
equation "d64 = wall * 0.4"
equation "pin_width = 8 mm"
equation "pin_thickness = 2.5 mm"
equation "pin_length = 6 mm"
equation "d69 = pin_thickness"
equation "d70 = pin_width"
equation "d72 = pin_width"
equation "d73 = pin_thickness"
equation "d75 = pin_width"
equation "d76 = pin_thickness"
equation "d78 = pin_thickness"
equation "d79 = pin_width"
equation "stem_height = bottom_height - 2 mm"
equation "d85 = wall"
equation "d87 = -overlap"
equation "d89 = -stem_height"
equation "d91 = -pin_length"
equation "hook_height = 2.7 mm"
equation "hook_depth = 0.8 mm"
equation "d95 = hook_depth"
equation "d96 = hook_height"
equation "d97 = hook_depth"
equation "d98 = hook_height"
equation "d99 = hook_height"
equation "d100 = hook_depth"
equation "d101 = hook_height"
equation "d102 = hook_depth"
equation "d103 = -pin_width"
equation "d105 = -pin_width"
equation "d107 = -pin_width"
equation "d109 = -pin_width"
equation "d112 = wall"
equation "d113 = tol"
equation "d114 = tol"
equation "d115 = tol"
equation "d116 = tol"
equation "d117 = tol"
equation "d118 = tol"
equation "d119 = tol"
equation "d120 = tol"
equation "d121 = tol"
equation "d122 = tol"
equation "d123 = tol"
equation "d124 = tol"
equation "d125 = tol"
equation "d126 = tol"
equation "d127 = tol"
equation "d128 = tol"
equation "hook_depression_top = 0.2 mm"
equation "hook_depression_bottom = hook_depth + 0.2 mm"
equation "d131 = -hook_depression_bottom"
equation "d133 = -hook_depression_top"
equation "d135 = -hook_depression_bottom"
equation "d137 = -hook_depression_top"
equation "d139 = -hook_depression_bottom"
equation "d141 = -hook_depression_top"
equation "d143 = -hook_depression_bottom"
equation "d145 = -hook_depression_top"
equation "tol_rad = 0.5 mm"
named bodies: "PCB"
